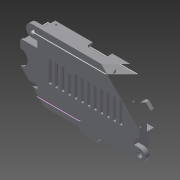
# Autodesk Inventor part: RaspiCaseLower
Saved by Autodesk Inventor 2014 SP1 (Build 180222100, 222)
## iProperties
Created: 2014-02-10
Part Number: RaspiCaseLower
Material: Generic
Document SubType Name: Modeling
Designer: Jack
Density: 1 g/cm^3
Appearance: Default
Author: Jack
Autodesk Inventor part; units mm, degrees
ref_plane "YZ Plane" through (0, 0, 0) normal (1, 0, 0) x (0, 1, 0)
ref_plane "XZ Plane" through (0, 0, 0) normal (0, 1, 0) x (-1, 0, 0)
ref_plane "XY Plane" through (0, 0, 0) normal (0, 0, 1) x (1, 0, 0)
sketch "Sketch1" plane through (0, 0, 0) normal (0, 1, 0) x (-1, 0, 0)
  line L0 (0, 0) -> (90, 0)
  line L1 (90, 0) -> (90, 61)
  line L2 (90, 61) -> (0, 61)
  line L3 (0, 61) -> (0, 0)
  dimension "d0" = 90
  dimension "d1" = 61
  constraints: 8 end point, 2 perpendicular, 1 horizontal, 1 parallel
  measures "d0" distance of L0.start L0.end
  measures "d1" distance of L0.end L1.end
extrude "Extrusion1" add sketch "Sketch1" along normal blind 2
sketch "Sketch2" plane through (0, 2, 0) normal (0, 1, 0) x (1, 0, 0)
  line L0 (0, 0) -> (-90, 0) projected
  line L1 (-90, 0) -> (-90, -61) projected
  line L2 (-90, -61) -> (0, -61) projected
  line L3 (0, -61) -> (0, 0) projected
  line L4 (-88, -2) -> (-2, -2)
  line L5 (-2, -2) -> (-2, -59)
  line L6 (-2, -59) -> (-88, -59)
  line L7 (-88, -59) -> (-88, -2)
  dimension "d4" = 2
  constraints: 8 end point, 3 other
  measures "d4" distance between parallel lines of L0 L4
extrude "Extrusion2" add sketch "Sketch2" along normal blind 11.6
sketch "Sketch3" plane through (0, 2, 0) normal (0, 1, 0) x (1, 0, 0)
  line L0 (-2, -59) -> (-2, -2) projected
  line L1 (-2, -2) -> (-88, -2) projected
  line L2 (-88, -2) -> (-88, -59) projected
  line L3 (-88, -59) -> (-2, -59) projected
  line L4 (-86, -4) -> (-4, -4)
  line L5 (-4, -4) -> (-4, -57)
  line L6 (-4, -57) -> (-86, -57)
  line L7 (-86, -57) -> (-86, -4)
  point P0 (0, 0)
  dimension "d7" = 2
  constraints: 8 end point, 3 other
  measures "d7" distance between parallel lines of L1 L4
extrude "Extrusion3" add sketch "Sketch3" along normal blind 2
sketch "Sketch4" plane through (-90, 0, 61) normal (0, 0, 1) x (1, 0, 0)
  line L0 (0, 13.6) -> (90, 13.6) projected
  line L1 (0, 0) -> (0, 13.6) projected
  line L2 (38, 13.6) -> (38, 7.1)
  line L3 (56.2, 13.6) -> (56.2, 7.1)
  line L4 (38, 7.1) -> (56.2, 7.1)
  dimension "d10" = 38
  dimension "d11" = 56.2
  dimension "d12" = 6.5
  constraints: 6 end point, 3 parallel, 2 point on line, 1 perpendicular
  measures "d10" distance between parallel lines of L1 L2
  measures "d11" distance between parallel lines of L1 L3
  measures "d12" distance of L2.start L2.end
extrude "Extrusion4" cut sketch "Sketch4" against normal blind 2
chamfer "Chamfer1" distance 2 angle 45 2 edges at (-52, 7.1, 60) (-33.8, 7.1, 60)
sketch "Sketch5" plane through (0, 0, 61) normal (1, 0, 0) x (0, 0, -1)
  line L0 (0, 13.6) -> (61, 13.6) projected
  line L1 (0, 0) -> (0, 13.6) projected
  line L2 (3.8, 13.6) -> (3.8, 7.1)
  line L3 (20.7, 13.6) -> (20.7, 7.1)
  line L4 (3.8, 7.1) -> (20.7, 7.1)
  dimension "d18" = 16.9
  dimension "d19" = 3.8
  dimension "d20" = 6.5
  constraints: 6 end point, 3 parallel, 2 point on line, 1 perpendicular
  measures "d18" distance between parallel lines of L2 L3
  measures "d19" distance between parallel lines of L1 L2
  measures "d20" distance of L2.start L2.end
extrude "Extrusion5" cut sketch "Sketch5" against normal blind 2
sketch "Sketch6" plane through (0, 13.6, 0) normal (0, 1, 0) x (1, 0, 0)
  line L0 (0, -40.3) -> (0, 0) projected
  line L1 (-2, -2) -> (-2, -40.3) projected
  line L2 (0, -57.2) -> (-2, -57.2) projected
  line L3 (-2, -57.2) -> (-2, -59) projected
  line L4 (-2, -59) -> (-33.8, -59) projected
  line L5 (-33.8, -59) -> (-33.8, -61) projected
  line L6 (-33.8, -61) -> (0, -61) projected
  line L7 (0, -61) -> (0, -57.2) projected
  line L8 (0, -40.3) -> (0, -57.2) projected
  line L9 (0, -40.3) -> (-2, -40.3) projected
  line L10 (-2, -57.2) -> (-2, -40.3) projected
  line L11 (0, -57.2) -> (-2, -57.2) projected
  line L12 (-2, -34.7) -> (5, -34.7) construction
  line L13 (5, -34.7) -> (5, -35.9)
  line L14 (5, -35.9) -> (5, -19.7)
  line L15 (5, -19.7) -> (0, -14.7)
  line L16 (0, -14.7) -> (0, -40.3)
  line L17 (0, -40.3) -> (0.6, -40.3)
  line L18 (5, -35.9) -> (0.6, -40.3)
  dimension "d24" = 7
  dimension "d26" = 16.2
  dimension "d27" = 135
  dimension "d131" = 14.7
  constraints: 14 end point, 2 parallel, 2 perpendicular, 2 point on line, 1 collinear, 1 horizontal
  measures "d24" distance of L12.start L12.end
  measures "d26" distance of L13.end L14.end
  measures "d27" angle of L14 L15
  measures "d131" distance of L0.end L15.end
extrude "Extrusion6" add sketch "Sketch6" against normal blind 13.6 contours L0 L15 L14 L13 L18 L17
sketch "Sketch7" plane through (5, 13.6, 35.9) normal (1, 0, 0) x (0, 0, -1)
  line L0 (0, 0) -> (16.2, 0) projected
  line L1 (-4.4, -6.5) -> (-21.3, -6.5) projected
  line L2 (-21.3, -6.5) -> (-21.3, 0) projected
  line L3 (-25.1, 0) -> (-21.3, 0) projected
  line L4 (-25.1, -13.6) -> (-25.1, 0) projected
  line L5 (-25.1, -13.6) -> (-4.4, -13.6) projected
  line L6 (0.95, 0) -> (0.95, -6.5)
  line L7 (0.95, -6.5) -> (15.25, -6.5)
  line L8 (15.25, -6.5) -> (15.25, 0)
  line L9 (16.2, 0) -> (16.2, -13.6) projected
  line L10 (21.2, 0) -> (21.2, -13.6) projected
  line L11 (21.2, -13.6) -> (35.9, -13.6) projected
  line L12 (35.9, -13.6) -> (35.9, 0) projected
  line L13 (21.2, 0) -> (35.9, 0) projected
  line L14 (-4.4, -13.6) -> (-4.4, -6.5) projected
  dimension "d30" = 14.3
  dimension "d32" = 6.5
  dimension "d130" = 0.95
  constraints: 6 end point, 2 perpendicular, 2 point on line, 1 parallel
  measures "d30" distance between parallel lines of L8 L6
  measures "d32" distance of L6.start L6.end
  measures "d130" distance between parallel lines of L9 L8
extrude "Extrusion7" cut sketch "Sketch7" against normal blind 7 contours L0 L8 L7 L6
sketch "Sketch8" plane through (0, 0, 0) normal (0, 0, -1) x (-1, 0, 0)
  line L0 (0, 13.6) -> (90, 13.6) projected
  line L1 (0, 0) -> (0, 13.6) projected
  circle A0 centre (24, 13.6) radius 4
  dimension "d35" = 8
  dimension "d36" = 24
  constraints: 1 centre point, 1 point on line
  measures "d35" diameter of A0
  measures "d36" distance from line of L1 A0.centre
extrude "Extrusion8" cut sketch "Sketch8" against normal blind 2
sketch "Sketch9" plane through (0, 13.6, 0) normal (0, 1, 0) x (1, 0, 0)
  line L0 (-28, 0) -> (-90, 0) projected
  line L1 (-20, 0) -> (-20, -2) projected
  line L2 (-20, -2) -> (-2, -2) projected
  line L3 (-2, -2) -> (-2, -20.65) projected
  line L4 (-2, -20.65) -> (5, -20.65) projected
  line L5 (5, -20.65) -> (5, -19.7) projected
  line L6 (5, -19.7) -> (0, -14.7) projected
  line L7 (0, -14.7) -> (0, 0) projected
  line L8 (0, 0) -> (-20, 0) projected
  line L9 (-32, 0) -> (-35, 5)
  line L10 (-35, 5) -> (-49, 5)
  line L11 (-49, 5) -> (-52, 0)
  dimension "d41" = 32
  dimension "d42" = 5
  dimension "d43" = 14
  dimension "d83" = 3
  dimension "d84" = 3
  constraints: 6 end point, 2 point on line, 1 parallel
  measures "d41" distance of point (0, 0) L9.start
  measures "d42" distance from line of L0 L9.end
  measures "d43" distance of L9.end L10.end
  measures "d83" horizontal distance of L9.end L9.start
  measures "d84" horizontal distance of L10.end L11.end
extrude "Extrusion9" add sketch "Sketch9" against normal blind 13.6 contours L0 L11 L10 L9
sketch "Sketch10" plane through (-35, 13.6, -5) normal (0, 0, -1) x (-1, 0, 0)
  line L0 (0, 0) -> (14, 0) projected
  line L1 (14, 0) -> (14, -13.6) projected
  circle A0 centre (7, 0) radius 5.5
  point P0 (-35, -13.6)
  dimension "d47" = 11
  dimension "d48" = 0
  dimension "d49" = 7
  constraints: 1 centre point
  measures "d47" diameter of A0
  measures "d48" distance from line of L0 A0.centre
  measures "d49" distance from line of L1 A0.centre
extrude "Extrusion10" cut sketch "Sketch10" against normal blind 9
sketch "Sketch11" plane through (-90, 0, 0) normal (-1, 0, 0) x (0, 0, 1)
  line L0 (0, 13.6) -> (61, 13.6) projected
  line L1 (0, 0) -> (0, 13.6) projected
  line L2 (9, 13.6) -> (9, 7.1)
  line L3 (9, 7.1) -> (56, 7.1)
  line L4 (56, 7.1) -> (56, 13.6)
  dimension "d52" = 47
  dimension "d53" = 9
  dimension "d54" = 6.5
  constraints: 6 end point, 2 perpendicular, 2 point on line, 1 parallel
  measures "d52" distance of L2.end L3.end
  measures "d53" distance between parallel lines of L1 L2
  measures "d54" distance of L2.start L2.end
extrude "Extrusion11" cut sketch "Sketch11" against normal blind 2
sketch "Sketch12" plane through (-90, 0, 0) normal (-1, 0, 0) x (0, 0, 1)
  line L0 (9, 7.1) -> (9, 13.6) projected
  line L1 (56, 7.1) -> (9, 7.1) projected
  line L2 (16.2, 7.1) -> (16.2, 2)
  line L3 (16.2, 2) -> (42, 2)
  line L4 (42, 2) -> (42, 7.1)
  dimension "d57" = 7.2
  dimension "d58" = 25.8
  dimension "d59" = 5.1
  constraints: 6 end point, 3 perpendicular, 2 point on line
  measures "d57" distance between parallel lines of L0 L2
  measures "d58" distance between parallel lines of L4 L2
  measures "d59" distance of L2.start L2.end
extrude "Extrusion12" cut sketch "Sketch12" against normal blind 4
sketch "Sketch13" plane through (-90, 0, 0) normal (-1, 0, 0) x (0, 0, 1)
  line L0 (16.2, 2) -> (16.2, 7.1) projected
  line L1 (16.2, 7.1) -> (9, 7.1) projected
  line L2 (0, 0) -> (61, 0) projected
  line L3 (56, 7.1) -> (42, 7.1) projected
  line L4 (42, 7.1) -> (42, 2) projected
  line L5 (42, 2) -> (16.2, 2) projected
  line L6 (14.2, 7.1) -> (14.2, 0)
  line L7 (44, 7.1) -> (44, 0)
  dimension "d62" = 2
  dimension "d63" = 2
  constraints: 4 end point, 4 point on line, 2 perpendicular
  measures "d62" distance between parallel lines of L0 L6
  measures "d63" distance between parallel lines of L7 L4
extrude "Extrusion13" add sketch "Sketch13" along normal blind 14
sketch "Sketch14" plane through (-104, 0, 0) normal (-1, 0, 0) x (0, 0, 1)
  line L0 (14.2, 7.1) -> (14.2, 0) projected
  line L1 (14.2, 0) -> (44, 0) projected
  line L2 (44, 0) -> (44, 7.1) projected
  line L3 (42, 2) -> (16.2, 2) projected
  line L4 (16.2, 2) -> (14.2, 2)
  line L5 (42, 2) -> (44, 2)
  point P0 (0, 0)
  constraints: 4 end point, 2 perpendicular, 2 point on line
extrude "Extrusion14" add sketch "Sketch14" along normal blind 2
fillet "Fillet1" radius 2 2 edges at (-106, 1, 14.2) (-106, 1, 44)
sketch "Sketch15" plane through (0, 2, 0) normal (0, 1, 0) x (1, 0, 0)
  line L0 (-106, -42) -> (-106, -16.2) projected
  circle A0 centre (-106, -29.1) radius 7
  point P0 (0, 0)
  dimension "d69" = 14
  constraints: 1 centre point, 1 midpoint
  measures "d69" diameter of A0
extrude "Extrusion15" cut sketch "Sketch15" against normal blind 2
sketch "Sketch16" plane through (0, 2, 0) normal (0, 1, 0) x (1, 0, 0)
  line L0 (-86, -57) -> (-4, -57) projected
  line L1 (-4, -57) -> (-4, -4) projected
  line L2 (-4, -4) -> (-86, -4) projected
  line L3 (-86, -4) -> (-86, -16.2) projected
  line L4 (-106, -22.1) -> (-106, -16.2) projected
  line L5 (-77, -9.5) -> (-72, -9.5)
  line L6 (-72, -9.5) -> (-72, -11)
  line L7 (-72, -11) -> (-77, -11)
  line L8 (-77, -11) -> (-77, -9.5)
  line L9 (-58, -10) -> (-58, -15)
  line L10 (-58, -15) -> (-53, -15)
  line L11 (-53, -15) -> (-53, -10)
  line L12 (-53, -10) -> (-58, -10)
  line L13 (-88, -16.2) -> (-86, -16.2) projected
  line L14 (-86, -16.2) -> (-86, -4) projected
  line L15 (-86, -4) -> (-4, -4) projected
  line L16 (-4, -4) -> (-4, -57) projected
  line L17 (-4, -57) -> (-86, -57) projected
  line L18 (-86, -57) -> (-86, -42) projected
  line L19 (-86, -42) -> (-88, -42) projected
  line L20 (-88, -59) -> (-88, -42) projected
  line L21 (-2, -59) -> (-88, -59) projected
  line L22 (-2, -2) -> (-2, -59) projected
  line L23 (-88, -2) -> (-2, -2) projected
  line L24 (-88, -16.2) -> (-88, -2) projected
  line L25 (-47, -2) -> (-47, -6)
  line L26 (-47, -6) -> (-43, -6)
  line L27 (-43, -6) -> (-43, -2)
  line L28 (-47, -2) -> (-43, -2)
  line L29 (-32, -6.5) -> (-32, -9.5)
  line L30 (-32, -9.5) -> (-30, -9.5)
  line L31 (-30, -9.5) -> (-30, -6.5)
  line L32 (-30, -6.5) -> (-32, -6.5)
  line L33 (-2, -17.8) -> (-6, -17.8)
  line L34 (-6, -17.8) -> (-6, -14.8)
  line L35 (-6, -14.8) -> (-2, -14.8)
  line L36 (-2, -14.8) -> (-2, -17.8)
  line L37 (-2, -37.5) -> (-6, -37.5)
  line L38 (-6, -37.5) -> (-6, -40.5)
  line L39 (-6, -40.5) -> (-2, -40.5)
  line L40 (-2, -37.5) -> (-2, -40.5)
  line L41 (-2, -55) -> (-6, -55)
  line L42 (-6, -55) -> (-6, -59)
  line L43 (-22.5, -59) -> (-22.5, -55)
  line L44 (-22.5, -55) -> (-26.5, -55)
  line L45 (-26.5, -55) -> (-26.5, -59)
  line L46 (-62.5, -59) -> (-62.5, -55)
  line L47 (-62.5, -55) -> (-66.5, -55)
  line L48 (-66.5, -55) -> (-66.5, -59)
  line L49 (-53, -52) -> (-58, -52)
  line L50 (-58, -52) -> (-58, -47)
  line L51 (-58, -47) -> (-53, -47)
  line L52 (-53, -47) -> (-53, -52)
  line L53 (-30, -49) -> (-32, -49)
  line L54 (-32, -49) -> (-32, -46)
  line L55 (-32, -46) -> (-30, -46)
  line L56 (-30, -46) -> (-30, -49)
  line L57 (-72, -47) -> (-77, -47)
  line L58 (-77, -47) -> (-77, -45.5)
  line L59 (-77, -45.5) -> (-72, -45.5)
  line L60 (-72, -45.5) -> (-72, -47)
  line L61 (-2, -4) -> (-6, -4)
  line L62 (-6, -4) -> (-6, -2)
  point P0 (0, 0)
  dimension "d72" = 5
  dimension "d73" = 1.5
  dimension "d74" = 5.5
  dimension "d75" = 9
  dimension "d76" = 5
  dimension "d77" = 5
  dimension "d78" = 6
  dimension "d79" = 28
  dimension "d80" = 4
  dimension "d81" = 4
  dimension "d82" = 39
  dimension "d85" = 3
  dimension "d86" = 2
  dimension "d87" = 26
  dimension "d88" = 2.5
  dimension "d89" = 4
  dimension "d90" = 3
  dimension "d91" = 10.8
  dimension "d92" = 4
  dimension "d93" = 3
  dimension "d94" = 16.5
  dimension "d95" = 4
  dimension "d96" = 4
  dimension "d97" = 4
  dimension "d98" = 4
  dimension "d99" = 16.5
  dimension "d100" = 4
  dimension "d101" = 4
  dimension "d102" = 36
  dimension "d103" = 5
  dimension "d104" = 5
  dimension "d105" = 5
  dimension "d106" = 1.5
  dimension "d107" = 3
  dimension "d108" = 2
  dimension "d109" = 4
  dimension "d110" = 2
  dimension "d112" = 8
  dimension "d113" = 5
  dimension "d114" = 10
  constraints: 92 end point, 23 perpendicular, 17 parallel, 14 point on line, 3 collinear, 3 horizontal, 3 vertical alignment
  measures "d72" distance of L5.start L5.end
  measures "d73" distance of L5.end L6.end
  measures "d74" distance between parallel lines of L2 L5
  measures "d75" distance between parallel lines of L3 L8
  measures "d76" distance of L9.start L9.end
  measures "d77" distance of L9.end L10.end
  measures "d78" distance between parallel lines of L2 L12
  measures "d79" distance between parallel lines of L3 L9
  measures "d80" distance of L25.start L25.end
  measures "d81" distance of L25.end L26.end
  measures "d82" distance between parallel lines of L14 L25
  measures "d85" distance of L29.start L29.end
  measures "d86" distance of L29.end L30.end
  measures "d87" distance between parallel lines of L1 L31
  measures "d88" distance between parallel lines of L2 L32
  measures "d89" distance of L33.start L33.end
  measures "d90" distance of L33.end L34.end
  measures "d91" distance between parallel lines of L15 L35
  measures "d92" distance of L37.start L37.end
  measures "d93" distance of L37.end L38.end
  measures "d94" distance between parallel lines of L0 L39
  measures "d95" distance of L41.start L41.end
  measures "d96" distance of L41.end L42.end
  measures "d97" distance of L43.start L43.end
  measures "d98" distance of L43.end L44.end
  measures "d99" distance between parallel lines of L42 L43
  measures "d100" distance of L46.start L46.end
  measures "d101" distance of L46.end L47.end
  measures "d102" distance between parallel lines of L45 L46
  measures "d103" distance of L49.start L49.end
  measures "d104" distance of L51.end L49.start
  measures "d105" distance of L57.start L57.end
  measures "d106" distance of L59.end L57.start
  measures "d107" distance of L55.end L53.start
  measures "d108" distance of L53.start L53.end
  measures "d109" distance of L61.start L61.end
  measures "d110" distance of L61.end L62.end
  measures "d112" distance between parallel lines of L0 L53
  measures "d113" distance between parallel lines of L17 L49
  measures "d114" distance between parallel lines of L17 L57
extrude "Extrusion16" add sketch "Sketch16" along normal blind 3.6 contours L48 L47 L46 L0 | L0 L46 L21 L48 | L45 L44 L43 L0 | L0 L43 L21 L45 | L42 L41 L1 L0 | L0 L1 L41 L22 L21 L42 | L39 L38 L37 L1 | L1 L37 L22 L39 | L33 L34 L35 L1 | L1 L35 L22 L33 | L2 L62 L23 L22 L61 | L27 L26 L25 L2 | L2 L25 L23 L27 | L5 L6 L7 L8 | L12 L11 L10 L9 | L32 L31 L30 L29 | L49 L50 L51 L52 | L53 L54 L55 L56 | L57 L58 L59 L60
sketch "Sketch17" plane through (0, 2, 0) normal (0, 1, 0) x (1, 0, 0)
  line L0 (-22.5, -57) -> (-6, -57) projected
  line L1 (-4, -37.5) -> (-4, -17.8) projected
  line L2 (-11, -40.75) -> (-13.5, -40.75)
  line L3 (-13.5, -40.75) -> (-13.5, -20.75)
  line L4 (-13.5, -20.75) -> (-11, -20.75)
  line L5 (-11, -20.75) -> (-11, -40.75)
  line L6 (-17, -40.75) -> (-19.5, -40.75)
  line L7 (-19.5, -40.75) -> (-19.5, -20.75)
  line L8 (-19.5, -20.75) -> (-17, -20.75)
  line L9 (-17, -20.75) -> (-17, -40.75)
  line L10 (-23, -40.75) -> (-25.5, -40.75)
  line L11 (-25.5, -40.75) -> (-25.5, -20.75)
  line L12 (-25.5, -20.75) -> (-23, -20.75)
  line L13 (-23, -20.75) -> (-23, -40.75)
  line L14 (-29, -40.75) -> (-31.5, -40.75)
  line L15 (-31.5, -40.75) -> (-31.5, -20.75)
  line L16 (-31.5, -20.75) -> (-29, -20.75)
  line L17 (-29, -20.75) -> (-29, -40.75)
  line L18 (-35, -40.75) -> (-37.5, -40.75)
  line L19 (-37.5, -40.75) -> (-37.5, -20.75)
  line L20 (-37.5, -20.75) -> (-35, -20.75)
  line L21 (-35, -20.75) -> (-35, -40.75)
  line L22 (-41, -40.75) -> (-43.5, -40.75)
  line L23 (-43.5, -40.75) -> (-43.5, -20.75)
  line L24 (-43.5, -20.75) -> (-41, -20.75)
  line L25 (-41, -20.75) -> (-41, -40.75)
  line L26 (-47, -40.75) -> (-49.5, -40.75)
  line L27 (-49.5, -40.75) -> (-49.5, -20.75)
  line L28 (-49.5, -20.75) -> (-47, -20.75)
  line L29 (-47, -20.75) -> (-47, -40.75)
  line L30 (-53, -40.75) -> (-55.5, -40.75)
  line L31 (-55.5, -40.75) -> (-55.5, -20.75)
  line L32 (-55.5, -20.75) -> (-53, -20.75)
  line L33 (-53, -20.75) -> (-53, -40.75)
  line L34 (-59, -40.75) -> (-61.5, -40.75)
  line L35 (-61.5, -40.75) -> (-61.5, -20.75)
  line L36 (-61.5, -20.75) -> (-59, -20.75)
  line L37 (-59, -20.75) -> (-59, -40.75)
  line L38 (-65, -40.75) -> (-67.5, -40.75)
  line L39 (-67.5, -40.75) -> (-67.5, -20.75)
  line L40 (-67.5, -20.75) -> (-65, -20.75)
  line L41 (-65, -20.75) -> (-65, -40.75)
  line L42 (-71, -40.75) -> (-73.5, -40.75)
  line L43 (-73.5, -40.75) -> (-73.5, -20.75)
  line L44 (-73.5, -20.75) -> (-71, -20.75)
  line L45 (-71, -20.75) -> (-71, -40.75)
  line L46 (-77, -40.75) -> (-79.5, -40.75)
  line L47 (-79.5, -40.75) -> (-79.5, -20.75)
  line L48 (-79.5, -20.75) -> (-77, -20.75)
  line L49 (-77, -20.75) -> (-77, -40.75)
  point P0 (0, 0)
  dimension "d117" = 2.5
  dimension "d118" = 20
  dimension "d119" = 7
  dimension "d120" = 16.25
  dimension "d123" = 6
  constraints: 96 end point, 2 horizontal, 2 parallel, 1 collinear, 1 perpendicular, 87 other
  measures "d117" distance of L3.end L4.end
  measures "d118" distance of L2.end L3.end
  measures "d119" distance between parallel lines of L1 L5
  measures "d120" distance between parallel lines of L0 L2
  measures "d123" distance of L2.start L6.start
extrude "Extrusion17" cut sketch "Sketch17" against normal blind 2
sketch "Sketch18" plane through (0, 2, 0) normal (0, 1, 0) x (1, 0, 0)
  line L0 (-4, -14.8) -> (-4, -4) projected
  line L1 (-4, -4) -> (-43, -4) projected
  line L2 (-86, -42) -> (-86, -57) projected
  line L3 (-86, -57) -> (-66.5, -57) projected
  circle A0 centre (-62, -40.5) radius 3
  circle A1 centre (-7.5, -15) radius 3
  point P0 (0, 0)
  dimension "d132" = 16.5
  dimension "d133" = 24
  dimension "d134" = 3.5
  dimension "d135" = 11
  dimension "d136" = 6
  dimension "d137" = 6
  constraints: 2 centre point
  measures "d132" distance from line of L3 A0.centre
  measures "d133" distance from line of A0.centre L2
  measures "d134" distance from line of L0 A1.centre
  measures "d135" distance from line of L1 A1.centre
  measures "d136" diameter of A0
  measures "d137" diameter of A1
extrude "Extrusion18" add sketch "Sketch18" along normal blind 3.6
sketch "Sketch19" plane through (-7.5, 5.6, 15) normal (0, 1, 0) x (-0.4708383, 0, 0.8822196)
  circle A0 centre (0, 0) radius 3 projected
  circle A1 centre (0, 0) radius 0.75
  point P0 (-16.7646, -0.4459)
  dimension "d140" = 1.5
  constraints: 1 centre point, 1 coincident
  measures "d140" diameter of A1
extrude "Extrusion19" cut sketch "Sketch19" against normal blind 3.5 contours A1
sketch "Sketch20" plane through (-62, 5.6, 40.5) normal (0, 1, 0) x (1, 0, 0)
  circle A0 centre (0, 0) radius 3 projected
  circle A1 centre (0, 0) radius 0.75
  point P0 (62, 40.5)
  dimension "d143" = 1.5
  constraints: 1 centre point, 1 coincident
  measures "d143" diameter of A1
extrude "Extrusion20" cut sketch "Sketch20" against normal blind 3.5 contours A1
sketch "Sketch22" plane through (0, 2, 0) normal (0, -1, 0) x (1, 0, 0)
  line L0 (-61.5, 40.75) -> (-61.5, 37.542) projected
  arc A0 (-61.5, 37.542) -> (-59, 40.5) centre (-62, 40.5) ccw projected
  arc A1 (-59, 40.5) -> (-59.0104, 40.75) centre (-62, 40.5) ccw projected
  line L1 (-59.0104, 40.75) -> (-61.5, 40.75) projected
  point P0 (0, 0)
extrude "Extrusion22" add sketch "Sketch22" along normal up to surface (2 mm away)
sketch "Sketch24" plane through (-90, 0, 61) normal (0, 0, 1) x (1, 0, 0)
  line L0 (0, 13.6) -> (38, 13.6) projected
  line L1 (0, 0) -> (0, 13.6) projected
  circle A0 centre (7, 10.6) radius 0.75
  dimension "d155" = 1.5
  dimension "d156" = 7
  dimension "d157" = 3
  constraints: 1 centre point
  measures "d155" diameter of A0
  measures "d156" distance from line of L1 A0.centre
  measures "d157" distance from line of L0 A0.centre
extrude "Extrusion24" cut sketch "Sketch24" against normal blind 2
sketch "Sketch25" plane through (0, 0, 0) normal (0, 0, -1) x (-1, 0, 0)
  line L0 (0, 13.6) -> (20, 13.6) projected
  line L1 (0, 0) -> (0, 13.6) projected
  circle A0 centre (7, 10.6) radius 0.75
  dimension "d160" = 1.5
  dimension "d161" = 7
  dimension "d162" = 3
  constraints: 1 centre point
  measures "d160" diameter of A0
  measures "d161" distance from line of L1 A0.centre
  measures "d162" distance from line of L0 A0.centre
extrude "Extrusion25" cut sketch "Sketch25" against normal blind 2
ref_plane "Work Plane1" through (-90, 0, 55.5) normal (0, 0, 1) x (1, 0, 0)
ref_plane "Work Plane2" through (-90, 0, 5.5) normal (0, 0, -1) x (-1, 0, 0)
sketch "Sketch26" plane through (0, 0, 0) normal (0, -1, 0) x (1, 0, 0)
  line L0 (-90, 0) -> (-90, 14.2) projected
  line L1 (0, 14.7) -> (0, 0) projected
  line L2 (0, 61) -> (0, 40.3) projected
  line L3 (-90, 44) -> (-90, 61) projected
  line L4 (-128.6971, 55.5) -> (27.2828, 55.5) projected
  line L5 (27.2828, 5.5) -> (-128.6971, 5.5) projected
  circle A0 centre (-95, 55.5) radius 2.5 construction
  circle A1 centre (-95, 5.5) radius 2.5 construction
  circle A2 centre (5, 55.5) radius 2.5 construction
  circle A3 centre (5, 5.5) radius 2.5 construction
  arc A4 (-95, 11) -> (-95, 0) centre (-95, 5.5) ccw
  arc A5 (-95, 61) -> (-95, 50) centre (-95, 55.5) ccw
  arc A6 (5, 50) -> (5, 61) centre (5, 55.5) ccw
  arc A7 (5, 0) -> (5, 11) centre (5, 5.5) ccw
  line L6 (5, 61) -> (0, 61)
  line L7 (5, 50) -> (0, 50)
  line L8 (5, 11) -> (0, 11)
  line L9 (5, 0) -> (0, 0)
  line L10 (-95, 11) -> (-90, 11)
  line L11 (-95, 0) -> (-90, 0)
  line L12 (-95, 50) -> (-90, 50)
  line L13 (-95, 61) -> (-90, 61)
  dimension "d167" = 5
  dimension "d168" = 5
  dimension "d169" = 5
  dimension "d170" = 5
  dimension "d171" = 5
  dimension "d172" = 5
  dimension "d173" = 5
  dimension "d174" = 5
  dimension "d175" = 11
  dimension "d176" = 11
  dimension "d177" = 11
  dimension "d178" = 11
  constraints: 16 end point, 8 centre point, 8 point on circle, 8 point on line, 8 tangent, 4 coincident, 4 perpendicular
  measures "d167" diameter of A0
  measures "d168" diameter of A1
  measures "d169" diameter of A2
  measures "d170" diameter of A3
  measures "d171" distance from line of L3 A0.centre
  measures "d172" distance from line of L0 A1.centre
  measures "d173" distance from line of L1 A3.centre
  measures "d174" distance from line of L2 A2.centre
  measures "d175" diameter of A4
  measures "d176" diameter of A5
  measures "d177" diameter of A6
  measures "d178" diameter of A7
extrude "Extrusion26" add sketch "Sketch26" against normal blind 4
hole "Hole1" at (5, 4, 55.5) direction (0, -1, 0) diameter 5 end through all
hole "Hole2" at (5, 4, 5.5) direction (0, -1, 0) diameter 5 end through all
hole "Hole3" at (-95, 4, 55.5) direction (0, -1, 0) diameter 5 end through all
hole "Hole4" at (-95, 4, 5.5) direction (0, -1, 0) diameter 5 end through all
chamfer "Chamfer2" distance 3 angle 45 1 edges at (0, 8.8, 0)
chamfer "Chamfer3" distance 3 angle 45 1 edges at (0, 8.8, 61)
chamfer "Chamfer4" distance 3 angle 45 1 edges at (-90, 8.8, 61)
chamfer "Chamfer5" distance 3 angle 45 1 edges at (-90, 8.8, 0)
body "Solid1"
